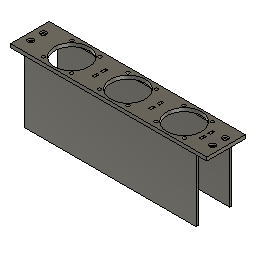
ducted_fan_plate (Autodesk Fusion 360 design; units mm, degrees)
part number: 2026-08-26-09-02-40-057
Autodesk Fusion 360 part; units mm, degrees
sketch "Plate" plane through (0, 0, 0) normal (0, 0, 1) x (1, 0, 0)
  line L0 (-111, 0.4) -> (111, 0.4)
  line L1 (111, 0.4) -> (111, 44.05)
  line L2 (111, 44.05) -> (-111, 44.05)
  line L3 (-111, 44.05) -> (-111, 0.4)
extrude "Plate (1)" add sketch "Plate" along normal blind 4
sketch "Duct walls" plane through (0, 0, 0) normal (0, 0, 1) x (1, 0, 0)
  line L0 (-97.22, 2.1) -> (97.22, 2.1)
  line L1 (97.22, 2.1) -> (97.22, 4.3)
  line L2 (97.22, 4.3) -> (-97.22, 4.3)
  line L3 (-97.22, 4.3) -> (-97.22, 2.1)
  line L4 (-97.22, 40.15) -> (97.22, 40.15)
  line L5 (97.22, 40.15) -> (97.22, 42.35)
  line L6 (97.22, 42.35) -> (-97.22, 42.35)
  line L7 (-97.22, 42.35) -> (-97.22, 40.15)
extrude "Duct walls (1)" add sketch "Duct walls" against normal blind 72
sketch "Openings and holes" plane through (0, 0, 0) normal (0, 0, 1) x (1, 0, 0)
  circle A0 centre (-63.55, 22.225) radius 19.5
  circle A1 centre (-79.55, 6.225) radius 1.8
  circle A2 centre (-79.55, 38.225) radius 1.8
  circle A3 centre (-47.55, 6.225) radius 1.8
  circle A4 centre (-47.55, 38.225) radius 1.8
  circle A5 centre (0, 22.225) radius 19.5
  circle A6 centre (-16, 6.225) radius 1.8
  circle A7 centre (-16, 38.225) radius 1.8
  circle A8 centre (16, 6.225) radius 1.8
  circle A9 centre (16, 38.225) radius 1.8
  circle A10 centre (63.55, 22.225) radius 19.5
  circle A11 centre (47.55, 6.225) radius 1.8
  circle A12 centre (47.55, 38.225) radius 1.8
  circle A13 centre (79.55, 6.225) radius 1.8
  circle A14 centre (79.55, 38.225) radius 1.8
  circle A15 centre (-102.82, 15) radius 1.7
  circle A16 centre (-102.82, 29.45) radius 1.7
  circle A17 centre (102.82, 15) radius 1.7
  circle A18 centre (102.82, 29.45) radius 1.7
extrude "Openings and holes (1)" cut sketch "Openings and holes" along normal blind 4
sketch "Tie slots" plane through (0, 0, 0) normal (0, 0, 1) x (1, 0, 0)
  line L0 (-33.03, 15) -> (-30.53, 15)
  line L1 (-30.53, 15) -> (-30.53, 20)
  line L2 (-30.53, 20) -> (-33.03, 20)
  line L3 (-33.03, 20) -> (-33.03, 15)
  line L4 (-33.03, 24.5) -> (-30.53, 24.5)
  line L5 (-30.53, 24.5) -> (-30.53, 29.5)
  line L6 (-30.53, 29.5) -> (-33.03, 29.5)
  line L7 (-33.03, 29.5) -> (-33.03, 24.5)
  line L8 (30.53, 15) -> (33.03, 15)
  line L9 (33.03, 15) -> (33.03, 20)
  line L10 (33.03, 20) -> (30.53, 20)
  line L11 (30.53, 20) -> (30.53, 15)
  line L12 (30.53, 24.5) -> (33.03, 24.5)
  line L13 (33.03, 24.5) -> (33.03, 29.5)
  line L14 (33.03, 29.5) -> (30.53, 29.5)
  line L15 (30.53, 29.5) -> (30.53, 24.5)
  line L16 (88.19, 15) -> (90.69, 15)
  line L17 (90.69, 15) -> (90.69, 20)
  line L18 (90.69, 20) -> (88.19, 20)
  line L19 (88.19, 20) -> (88.19, 15)
  line L20 (88.19, 24.5) -> (90.69, 24.5)
  line L21 (90.69, 24.5) -> (90.69, 29.5)
  line L22 (90.69, 29.5) -> (88.19, 29.5)
  line L23 (88.19, 29.5) -> (88.19, 24.5)
extrude "Tie slots (1)" cut sketch "Tie slots" along normal blind 4
ref_plane "WorkPlane1" through (0, 0, 4) normal (0, 0, 1) x (1, 0, 0)
sketch "Head counterbores" plane through (0, 0, 4) normal (0, 0, 1) x (1, 0, 0)
  circle A0 centre (-102.82, 15) radius 3.25
  circle A1 centre (-102.82, 29.45) radius 3.25
  circle A2 centre (102.82, 15) radius 3.25
  circle A3 centre (102.82, 29.45) radius 3.25
extrude "Head counterbores (1)" cut sketch "Head counterbores" against normal blind 2
named bodies: "Ducted Fan Plate"
